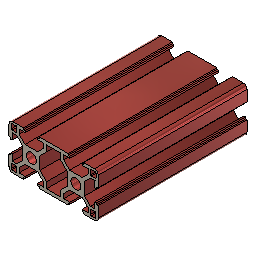
3060 Extrusion (Autodesk Fusion 360 design; units mm, degrees)
Autodesk Fusion 360 part; units mm, degrees
sketch "Sketch1" plane through (0, 0, 0) normal (0, 0, 1) x (1, 0, 0)
  circle A0 centre (10, 10) radius 2.5
  line L0 (13.9, 6.1) -> (6.1, 13.9) construction
  line L1 (0, 6.4) -> (0, 1.5)
  line L2 (4.5, 1.8) -> (6.9, 1.8)
  line L3 (3.5808, 4.5) -> (6.1, 7.0192)
  line L4 (4.5, 3.5808) -> (7.0192, 6.1)
  line L5 (0.5, 6.9) -> (0.5, 6.4)
  line L6 (0.5, 6.4) -> (0, 6.4)
  line L7 (6.9, 0) -> (6.4, 0) construction
  line L8 (6.4, 0) -> (6.4, 0.5)
  line L9 (6.4, 0.5) -> (6.9, 0.5)
  arc A1 (0, 1.5) -> (1.5, 0) centre (1.5, 1.5) ccw
  line L10 (1.8, 6.9) -> (0.5, 6.9)
  line L11 (1.8, 6.9) -> (1.8, 6.4)
  line L12 (1.8, 6.4) -> (1.8, 4.5)
  line L13 (3.5808, 4.5) -> (1.8, 4.5)
  line L14 (6.1, 10) -> (6.1, 7.0192)
  line L15 (7.0192, 6.1) -> (10, 6.1)
  line L16 (4.5, 1.8) -> (4.5, 3.5808)
  line L17 (6.9, 0.5) -> (6.9, 1.8)
  line L18 (1.5, 0) -> (6.4, 0)
  line L19 (6.4, 0) -> (6.9, 0)
  line L20 (0, 6.9) -> (0, 6.4)
  line L21 (10, 13.9) -> (10, 6.1) construction
  line L22 (13.9, 10) -> (6.1, 10) construction
  line L23 (20, 6.4) -> (19.5, 6.4)
  line L24 (19.5, 6.4) -> (19.5, 6.9)
  line L25 (19.5, 6.9) -> (18.2, 6.9)
  line L26 (18.2, 4.5) -> (18.2, 6.9)
  line L27 (18.2, 4.5) -> (16.4192, 4.5)
  line L28 (16.4192, 4.5) -> (13.9, 7.0192)
  line L29 (13.9, 7.0192) -> (13.9, 10)
  line L30 (15.5, 3.5808) -> (12.9808, 6.1)
  line L31 (15.5, 3.5808) -> (15.5, 1.8)
  line L32 (13.6, 1.8) -> (15.5, 1.8)
  line L33 (13.1, 1.8) -> (13.6, 1.8)
  line L34 (13.1, 1.8) -> (13.1, 0.5)
  line L35 (13.1, 0.5) -> (13.6, 0.5)
  line L36 (13.6, 0.5) -> (13.6, 0)
  line L37 (10, 6.1) -> (12.9808, 6.1)
  line L38 (13.6, 0) -> (18.5, 0)
  arc A2 (18.5, 0) -> (20, 1.5) centre (18.5, 1.5) ccw
  line L39 (20, 1.5) -> (20, 6.4)
  line L40 (13.6, 20) -> (13.6, 19.5)
  line L41 (13.6, 19.5) -> (13.1, 19.5)
  line L42 (13.1, 19.5) -> (13.1, 18.2)
  line L43 (15.5, 18.2) -> (13.1, 18.2)
  line L44 (15.5, 18.2) -> (15.5, 16.4192)
  line L45 (15.5, 16.4192) -> (12.9808, 13.9)
  line L46 (12.9808, 13.9) -> (10, 13.9)
  line L47 (16.4192, 15.5) -> (13.9, 12.9808)
  line L48 (16.4192, 15.5) -> (18.2, 15.5)
  line L49 (18.2, 13.6) -> (18.2, 15.5)
  line L50 (18.2, 13.1) -> (18.2, 13.6)
  line L51 (18.2, 13.1) -> (19.5, 13.1)
  line L52 (19.5, 13.1) -> (19.5, 13.6)
  line L53 (19.5, 13.6) -> (20, 13.6)
  line L54 (13.9, 10) -> (13.9, 12.9808)
  line L55 (20, 13.6) -> (20, 18.5)
  arc A3 (20, 18.5) -> (18.5, 20) centre (18.5, 18.5) ccw
  line L56 (18.5, 20) -> (13.6, 20)
  line L57 (0, 13.6) -> (0.5, 13.6)
  line L58 (0.5, 13.6) -> (0.5, 13.1)
  line L59 (0.5, 13.1) -> (1.8, 13.1)
  line L60 (1.8, 15.5) -> (1.8, 13.1)
  line L61 (1.8, 15.5) -> (3.5808, 15.5)
  line L62 (3.5808, 15.5) -> (6.1, 12.9808)
  line L63 (6.1, 12.9808) -> (6.1, 10)
  line L64 (4.5, 16.4192) -> (7.0192, 13.9)
  line L65 (4.5, 16.4192) -> (4.5, 18.2)
  line L66 (6.4, 18.2) -> (4.5, 18.2)
  line L67 (6.9, 18.2) -> (6.4, 18.2)
  line L68 (6.9, 18.2) -> (6.9, 19.5)
  line L69 (6.9, 19.5) -> (6.4, 19.5)
  line L70 (6.4, 19.5) -> (6.4, 20)
  line L71 (10, 13.9) -> (7.0192, 13.9)
  line L72 (6.4, 20) -> (1.5, 20)
  arc A4 (1.5, 20) -> (0, 18.5) centre (1.5, 18.5) ccw
  line L73 (0, 18.5) -> (0, 13.6)
  arc A5 (26, 1.5) -> (27.5, 0) centre (27.5, 1.5) ccw
  line L74 (41.5, 3.5808) -> (41.5, 1.8)
  line L75 (39.1, 19.5) -> (39.1, 18.2)
  line L76 (32.4, 20) -> (27.5, 20)
  line L77 (26, 6.9) -> (26, 6.4)
  line L78 (29.5808, 4.5) -> (32.1, 7.0192)
  line L79 (29.5808, 15.5) -> (32.1, 12.9808)
  line L80 (26, 13.6) -> (26.5, 13.6)
  line L81 (39.1, 0.5) -> (39.6, 0.5)
  line L82 (30.5, 16.4192) -> (30.5, 18.2)
  line L83 (27.8, 15.5) -> (27.8, 13.1)
  line L84 (36, 13.9) -> (36, 6.1) construction
  line L85 (32.4, 0) -> (32.4, 0.5)
  line L86 (39.6, 0.5) -> (39.6, 0)
  line L87 (32.1, 10) -> (32.1, 7.0192)
  line L88 (32.4, 19.5) -> (32.4, 20)
  line L89 (39.1, 1.8) -> (39.6, 1.8)
  line L90 (27.8, 6.9) -> (27.8, 6.4)
  line L91 (41.5, 16.4192) -> (38.9808, 13.9)
  line L92 (26.5, 13.1) -> (27.8, 13.1)
  line L93 (26.5, 6.4) -> (26, 6.4)
  line L94 (32.1, 12.9808) -> (32.1, 10)
  line L95 (27.5, 0) -> (32.4, 0)
  line L96 (32.9, 0.5) -> (32.9, 1.8)
  line L97 (32.9, 0) -> (32.4, 0) construction
  line L98 (30.5, 1.8) -> (30.5, 3.5808)
  line L99 (32.9, 19.5) -> (32.4, 19.5)
  line L100 (32.9, 18.2) -> (32.4, 18.2)
  line L101 (41.5, 18.2) -> (39.1, 18.2)
  line L102 (39.6, 19.5) -> (39.1, 19.5)
  line L103 (27.8, 6.9) -> (26.5, 6.9)
  line L104 (27.8, 15.5) -> (29.5808, 15.5)
  line L105 (36, 13.9) -> (33.0192, 13.9)
  line L106 (33.0192, 6.1) -> (36, 6.1)
  line L107 (41.5, 18.2) -> (41.5, 16.4192)
  line L108 (39.9, 10) -> (32.1, 10) construction
  line L109 (39.6, 1.8) -> (41.5, 1.8)
  line L110 (39.9, 6.1) -> (32.1, 13.9) construction
  line L111 (39.6, 0) -> (44.5, 0)
  line L112 (36, 6.1) -> (38.9808, 6.1)
  circle A6 centre (36, 10) radius 2.5
  line L113 (42.4192, 4.5) -> (39.9, 7.0192)
  line L114 (38.9808, 13.9) -> (36, 13.9)
  line L115 (41.5, 3.5808) -> (38.9808, 6.1)
  line L116 (39.9, 7.0192) -> (39.9, 10)
  line L117 (39.9, 10) -> (39.9, 12.9808)
  line L118 (30.5, 16.4192) -> (33.0192, 13.9)
  line L119 (42.4192, 15.5) -> (39.9, 12.9808)
  line L120 (26, 18.5) -> (26, 13.6)
  line L121 (39.6, 20) -> (39.6, 19.5)
  line L122 (32.4, 18.2) -> (30.5, 18.2)
  line L123 (26.5, 6.9) -> (26.5, 6.4)
  line L124 (39.1, 1.8) -> (39.1, 0.5)
  arc A7 (27.5, 20) -> (26, 18.5) centre (27.5, 18.5) ccw
  line L125 (44.5, 20) -> (39.6, 20)
  line L126 (26, 6.4) -> (26, 1.5)
  line L127 (30.5, 3.5808) -> (33.0192, 6.1)
  line L128 (32.4, 0) -> (32.9, 0)
  line L129 (32.4, 0.5) -> (32.9, 0.5)
  line L130 (29.5808, 4.5) -> (27.8, 4.5)
  line L131 (27.8, 6.4) -> (27.8, 4.5)
  line L132 (30.5, 1.8) -> (32.9, 1.8)
  line L133 (26.5, 13.6) -> (26.5, 13.1)
  line L134 (32.9, 18.2) -> (32.9, 19.5)
  line L135 (59.9, 6.1) -> (52.1, 13.9) construction
  circle A8 centre (56, 10) radius 2.5
  line L136 (56, 13.9) -> (56, 6.1) construction
  line L137 (66, 13.6) -> (66, 18.5)
  line L138 (61.5, 16.4192) -> (58.9808, 13.9)
  line L139 (59.9, 10) -> (59.9, 12.9808)
  line L140 (64.2, 13.1) -> (65.5, 13.1)
  line L141 (59.6, 20) -> (59.6, 19.5)
  line L142 (52.1, 12.9808) -> (52.1, 10)
  line L143 (59.1, 19.5) -> (59.1, 18.2)
  line L144 (64.2, 13.1) -> (64.2, 13.6)
  line L145 (64.2, 13.6) -> (64.2, 15.5)
  line L146 (59.9, 10) -> (52.1, 10) construction
  line L147 (65.5, 13.1) -> (65.5, 13.6)
  line L148 (64.5, 20) -> (59.6, 20)
  line L149 (49.5808, 15.5) -> (52.1, 12.9808)
  line L150 (52.4, 19.5) -> (52.4, 20)
  line L151 (62.4192, 15.5) -> (64.2, 15.5)
  line L152 (59.1, 0.5) -> (59.6, 0.5)
  line L153 (65.5, 13.6) -> (66, 13.6)
  line L154 (50.5, 16.4192) -> (53.0192, 13.9)
  line L155 (61.5, 18.2) -> (61.5, 16.4192)
  line L156 (53.0192, 6.1) -> (56, 6.1)
  line L157 (50.5, 16.4192) -> (50.5, 18.2)
  line L158 (52.4, 0.5) -> (52.9, 0.5)
  line L159 (59.1, 1.8) -> (59.6, 1.8)
  line L160 (49.5808, 4.5) -> (52.1, 7.0192)
  line L161 (50.5, 1.8) -> (50.5, 3.5808)
  line L162 (61.5, 3.5808) -> (61.5, 1.8)
  line L163 (56, 13.9) -> (53.0192, 13.9)
  line L164 (52.4, 0) -> (52.4, 0.5)
  line L165 (50.5, 3.5808) -> (53.0192, 6.1)
  line L166 (66, 1.5) -> (66, 6.4)
  line L167 (59.6, 1.8) -> (61.5, 1.8)
  arc A9 (66, 18.5) -> (64.5, 20) centre (64.5, 18.5) ccw
  line L168 (52.1, 10) -> (52.1, 7.0192)
  line L169 (64.2, 4.5) -> (62.4192, 4.5)
  line L170 (59.6, 19.5) -> (59.1, 19.5)
  line L171 (61.5, 18.2) -> (59.1, 18.2)
  line L172 (61.5, 3.5808) -> (58.9808, 6.1)
  line L173 (52.9, 0) -> (52.4, 0) construction
  line L174 (59.9, 7.0192) -> (59.9, 10)
  line L175 (52.4, 18.2) -> (50.5, 18.2)
  line L176 (59.6, 0.5) -> (59.6, 0)
  line L177 (52.9, 18.2) -> (52.4, 18.2)
  line L178 (66, 6.4) -> (65.5, 6.4)
  line L179 (56, 6.1) -> (58.9808, 6.1)
  line L180 (52.9, 18.2) -> (52.9, 19.5)
  line L181 (59.6, 0) -> (64.5, 0)
  line L182 (62.4192, 4.5) -> (59.9, 7.0192)
  arc A10 (64.5, 0) -> (66, 1.5) centre (64.5, 1.5) ccw
  line L183 (50.5, 1.8) -> (52.9, 1.8)
  line L184 (52.4, 20) -> (47.5, 20)
  line L185 (64.2, 4.5) -> (64.2, 6.9)
  line L186 (65.5, 6.4) -> (65.5, 6.9)
  line L187 (52.4, 0) -> (52.9, 0)
  line L188 (52.9, 19.5) -> (52.4, 19.5)
  line L189 (65.5, 6.9) -> (64.2, 6.9)
  line L190 (59.1, 1.8) -> (59.1, 0.5)
  line L191 (47.5, 0) -> (52.4, 0)
  line L192 (58.9808, 13.9) -> (56, 13.9)
  line L193 (62.4192, 15.5) -> (59.9, 12.9808)
  line L194 (52.9, 0.5) -> (52.9, 1.8)
  line L195 (44.5, 20) -> (47.5, 20)
  line L196 (44.5, 0) -> (47.5, 0)
  line L197 (41.5, 18.2) -> (42.8, 18.2) construction
  line L198 (42.8, 18.2) -> (49.2, 18.2)
  line L199 (49.2, 1.8) -> (42.8, 1.8)
  line L200 (42.4192, 15.5) -> (42.8, 15.8808)
  line L201 (49.5808, 15.5) -> (49.2, 15.8808)
  line L202 (49.5808, 4.5) -> (49.2, 4.1192)
  line L203 (42.4192, 4.5) -> (42.8, 4.1192)
  line L204 (42.8, 15.8808) -> (42.8, 18.2)
  line L205 (49.2, 18.2) -> (49.2, 15.8808)
  line L206 (49.2, 4.1192) -> (49.2, 1.8)
  line L207 (42.8, 1.8) -> (42.8, 4.1192)
  arc A11 (2.5, -14.9884) -> (0, -17.4884) centre (2.5, -17.4884) ccw
  circle A12 centre (15, -29.9884) radius 3.4
  line L208 (10.9, -15.9884) -> (10.9, -17.1884)
  line L209 (19.2444, -24.1884) -> (10.7556, -24.1884)
  line L210 (9.2, -25.744) -> (9.2, -34.2327)
  line L211 (10.7556, -35.7884) -> (19.2444, -35.7884)
  line L212 (20.8, -34.2327) -> (20.8, -25.744)
  line L213 (1, -25.8884) -> (2.2, -25.8884)
  line L214 (0, -24.7884) -> (0, -21.7384)
  line L215 (0, -24.7884) -> (1, -24.7884)
  line L216 (1, -25.8884) -> (1, -24.7884)
  line L217 (2.2, -25.8884) -> (2.2, -24.7884)
  line L218 (2.2, -24.7884) -> (2.2, -21.7384)
  line L219 (2.5, -14.9884) -> (9.8, -14.9884)
  line L220 (6.75, -17.1884) -> (10.9, -17.1884)
  line L221 (9.8, -15.9884) -> (10.9, -15.9884)
  line L222 (9.8, -15.9884) -> (9.8, -14.9884)
  line L223 (2.2, -21.7384) -> (5.1944, -21.7384)
  line L224 (6.75, -20.1827) -> (6.75, -17.1884)
  line L225 (0, -17.4884) -> (0, -21.7384)
  line L226 (10.7556, -24.1884) -> (6.75, -20.1827)
  line L227 (9.2, -25.744) -> (5.1944, -21.7384)
  line L228 (4.825, -20.1634) -> (2.075, -20.1634)
  line L229 (1.575, -19.6634) -> (1.575, -16.9134)
  line L230 (2.075, -16.4134) -> (4.825, -16.4134)
  line L231 (5.325, -16.9134) -> (5.325, -19.6634)
  arc A13 (2.075, -16.4134) -> (1.575, -16.9134) centre (2.075, -16.9134) ccw
  arc A14 (5.325, -16.9134) -> (4.825, -16.4134) centre (4.825, -16.9134) ccw
  arc A15 (4.825, -20.1634) -> (5.325, -19.6634) centre (4.825, -19.6634) ccw
  arc A16 (1.575, -19.6634) -> (2.075, -20.1634) centre (2.075, -19.6634) ccw
  line L232 (2.2, -38.2384) -> (2.2, -34.0884)
  line L233 (1, -34.0884) -> (2.2, -34.0884)
  line L234 (1, -35.1884) -> (1, -34.0884)
  line L235 (1, -35.1884) -> (0, -35.1884)
  line L236 (0, -42.4884) -> (0, -35.1884)
  arc A17 (0, -42.4884) -> (2.5, -44.9884) centre (2.5, -42.4884) ccw
  line L237 (2.5, -44.9884) -> (6.75, -44.9884)
  line L238 (9.8, -44.9884) -> (6.75, -44.9884)
  line L239 (9.8, -44.9884) -> (9.8, -43.9884)
  line L240 (10.9, -43.9884) -> (9.8, -43.9884)
  line L241 (10.9, -43.9884) -> (10.9, -42.7884)
  line L242 (10.9, -42.7884) -> (9.8, -42.7884)
  line L243 (9.8, -42.7884) -> (6.75, -42.7884)
  line L244 (6.75, -42.7884) -> (6.75, -39.794)
  line L245 (10.7556, -35.7884) -> (6.75, -39.794)
  line L246 (9.2, -34.2327) -> (5.1944, -38.2384)
  line L247 (5.1944, -38.2384) -> (2.2, -38.2384)
  arc A18 (1.425, -42.9134) -> (1.925, -43.4134) centre (1.925, -42.9134) ccw
  line L248 (1.425, -42.9134) -> (1.425, -40.1634)
  arc A19 (1.925, -39.6634) -> (1.425, -40.1634) centre (1.925, -40.1634) ccw
  line L249 (1.925, -39.6634) -> (4.675, -39.6634)
  arc A20 (5.175, -40.1634) -> (4.675, -39.6634) centre (4.675, -40.1634) ccw
  line L250 (5.175, -40.1634) -> (5.175, -42.9134)
  arc A21 (4.675, -43.4134) -> (5.175, -42.9134) centre (4.675, -42.9134) ccw
  line L251 (4.675, -43.4134) -> (1.925, -43.4134)
  line L252 (23.25, -42.7884) -> (19.1, -42.7884)
  line L253 (19.1, -43.9884) -> (19.1, -42.7884)
  line L254 (20.2, -43.9884) -> (19.1, -43.9884)
  line L255 (20.2, -43.9884) -> (20.2, -44.9884)
  line L256 (27.5, -44.9884) -> (20.2, -44.9884)
  arc A22 (27.5, -44.9884) -> (30, -42.4884) centre (27.5, -42.4884) ccw
  line L257 (30, -42.4884) -> (30, -38.2384)
  line L258 (30, -35.1884) -> (30, -38.2384)
  line L259 (30, -35.1884) -> (29, -35.1884)
  line L260 (29, -34.0884) -> (29, -35.1884)
  line L261 (29, -34.0884) -> (27.8, -34.0884)
  line L262 (27.8, -34.0884) -> (27.8, -35.1884)
  line L263 (27.8, -35.1884) -> (27.8, -38.2384)
  line L264 (27.8, -38.2384) -> (24.8056, -38.2384)
  line L265 (20.8, -34.2327) -> (24.8056, -38.2384)
  line L266 (19.2444, -35.7884) -> (23.25, -39.794)
  line L267 (23.25, -39.794) -> (23.25, -42.7884)
  arc A23 (27.925, -43.5634) -> (28.425, -43.0634) centre (27.925, -43.0634) ccw
  line L268 (27.925, -43.5634) -> (25.175, -43.5634)
  arc A24 (24.675, -43.0634) -> (25.175, -43.5634) centre (25.175, -43.0634) ccw
  line L269 (24.675, -43.0634) -> (24.675, -40.3134)
  arc A25 (25.175, -39.8134) -> (24.675, -40.3134) centre (25.175, -40.3134) ccw
  line L270 (25.175, -39.8134) -> (27.925, -39.8134)
  arc A26 (28.425, -40.3134) -> (27.925, -39.8134) centre (27.925, -40.3134) ccw
  line L271 (28.425, -40.3134) -> (28.425, -43.0634)
  line L272 (27.8, -21.7384) -> (27.8, -25.8884)
  line L273 (29, -25.8884) -> (27.8, -25.8884)
  line L274 (29, -24.7884) -> (29, -25.8884)
  line L275 (29, -24.7884) -> (30, -24.7884)
  line L276 (30, -17.4884) -> (30, -24.7884)
  arc A27 (30, -17.4884) -> (27.5, -14.9884) centre (27.5, -17.4884) ccw
  line L277 (27.5, -14.9884) -> (23.25, -14.9884)
  line L278 (20.2, -14.9884) -> (23.25, -14.9884)
  line L279 (20.2, -14.9884) -> (20.2, -15.9884)
  line L280 (19.1, -15.9884) -> (20.2, -15.9884)
  line L281 (19.1, -15.9884) -> (19.1, -17.1884)
  line L282 (19.1, -17.1884) -> (20.2, -17.1884)
  line L283 (20.2, -17.1884) -> (23.25, -17.1884)
  line L284 (23.25, -17.1884) -> (23.25, -20.1827)
  line L285 (19.2444, -24.1884) -> (23.25, -20.1827)
  line L286 (20.8, -25.744) -> (24.8056, -21.7384)
  line L287 (24.8056, -21.7384) -> (27.8, -21.7384)
  arc A28 (28.575, -17.0634) -> (28.075, -16.5634) centre (28.075, -17.0634) ccw
  line L288 (28.575, -17.0634) -> (28.575, -19.8134)
  arc A29 (28.075, -20.3134) -> (28.575, -19.8134) centre (28.075, -19.8134) ccw
  line L289 (28.075, -20.3134) -> (25.325, -20.3134)
  arc A30 (24.825, -19.8134) -> (25.325, -20.3134) centre (25.325, -19.8134) ccw
  line L290 (24.825, -19.8134) -> (24.825, -17.0634)
  arc A31 (25.325, -16.5634) -> (24.825, -17.0634) centre (25.325, -17.0634) ccw
  line L291 (25.325, -16.5634) -> (28.075, -16.5634)
  circle A32 centre (55, -29.9884) radius 3.4
  line L292 (59.1, -15.9884) -> (60.2, -15.9884)
  line L293 (59.1, -43.9884) -> (59.1, -42.7884)
  line L294 (50.9, -43.9884) -> (50.9, -42.7884)
  line L295 (50.9, -42.7884) -> (49.8, -42.7884)
  line L296 (49.8, -44.9884) -> (49.8, -43.9884)
  line L297 (60.8, -34.2327) -> (60.8, -25.744)
  line L298 (49.8, -15.9884) -> (49.8, -14.9884)
  line L299 (50.9, -15.9884) -> (50.9, -17.1884)
  line L300 (60.2, -17.1884) -> (63.25, -17.1884)
  line L301 (50.9, -43.9884) -> (49.8, -43.9884)
  line L302 (50.7556, -35.7884) -> (59.2444, -35.7884)
  line L303 (59.2444, -24.1884) -> (63.25, -20.1827)
  line L304 (59.1, -15.9884) -> (59.1, -17.1884)
  line L305 (59.2444, -35.7884) -> (63.25, -39.794)
  line L306 (60.2, -43.9884) -> (59.1, -43.9884)
  line L307 (49.8, -15.9884) -> (50.9, -15.9884)
  line L308 (59.1, -17.1884) -> (60.2, -17.1884)
  line L309 (60.2, -14.9884) -> (60.2, -15.9884)
  line L310 (60.2, -43.9884) -> (60.2, -44.9884)
  line L311 (59.2444, -24.1884) -> (50.7556, -24.1884)
  line L312 (63.25, -42.7884) -> (59.1, -42.7884)
  arc A33 (41.575, -19.6634) -> (42.075, -20.1634) centre (42.075, -19.6634) ccw
  line L313 (40, -17.4884) -> (40, -21.7384)
  line L314 (42.2, -24.7884) -> (42.2, -21.7384)
  line L315 (40, -24.7884) -> (41, -24.7884)
  line L316 (67.5, -44.9884) -> (60.2, -44.9884)
  line L317 (41, -25.8884) -> (42.2, -25.8884)
  arc A34 (42.075, -16.4134) -> (41.575, -16.9134) centre (42.075, -16.9134) ccw
  line L318 (44.825, -20.1634) -> (42.075, -20.1634)
  line L319 (42.2, -25.8884) -> (42.2, -24.7884)
  arc A35 (45.325, -16.9134) -> (44.825, -16.4134) centre (44.825, -16.9134) ccw
  line L320 (60.8, -34.2327) -> (64.8056, -38.2384)
  arc A36 (42.5, -14.9884) -> (40, -17.4884) centre (42.5, -17.4884) ccw
  line L321 (40, -24.7884) -> (40, -21.7384)
  line L322 (60.8, -25.744) -> (64.8056, -21.7384)
  line L323 (45.325, -16.9134) -> (45.325, -19.6634)
  line L324 (60.2, -14.9884) -> (63.25, -14.9884)
  line L325 (42.5, -14.9884) -> (49.8, -14.9884)
  line L326 (50.7556, -24.1884) -> (46.75, -20.1827)
  line L327 (41.575, -19.6634) -> (41.575, -16.9134)
  line L328 (49.8, -42.7884) -> (46.75, -42.7884)
  line L329 (46.75, -17.1884) -> (50.9, -17.1884)
  line L330 (49.2, -25.744) -> (45.1944, -21.7384)
  line L331 (46.75, -20.1827) -> (46.75, -17.1884)
  line L332 (49.8, -44.9884) -> (46.75, -44.9884)
  line L333 (50.7556, -35.7884) -> (46.75, -39.794)
  arc A37 (44.825, -20.1634) -> (45.325, -19.6634) centre (44.825, -19.6634) ccw
  line L334 (42.075, -16.4134) -> (44.825, -16.4134)
  line L335 (63.25, -39.794) -> (63.25, -42.7884)
  line L336 (41, -25.8884) -> (41, -24.7884)
  line L337 (49.2, -25.744) -> (49.2, -34.2327)
  line L338 (42.2, -21.7384) -> (45.1944, -21.7384)
  line L339 (42.2, -38.2384) -> (42.2, -34.0884)
  line L340 (41.425, -42.9134) -> (41.425, -40.1634)
  arc A38 (45.175, -40.1634) -> (44.675, -39.6634) centre (44.675, -40.1634) ccw
  arc A39 (41.425, -42.9134) -> (41.925, -43.4134) centre (41.925, -42.9134) ccw
  line L341 (41, -35.1884) -> (40, -35.1884)
  arc A40 (41.925, -39.6634) -> (41.425, -40.1634) centre (41.925, -40.1634) ccw
  line L342 (41.925, -39.6634) -> (44.675, -39.6634)
  line L343 (45.175, -40.1634) -> (45.175, -42.9134)
  line L344 (49.2, -34.2327) -> (45.1944, -38.2384)
  line L345 (67.5, -14.9884) -> (63.25, -14.9884)
  arc A41 (44.675, -43.4134) -> (45.175, -42.9134) centre (44.675, -42.9134) ccw
  arc A42 (40, -42.4884) -> (42.5, -44.9884) centre (42.5, -42.4884) ccw
  line L346 (41, -35.1884) -> (41, -34.0884)
  line L347 (41, -34.0884) -> (42.2, -34.0884)
  line L348 (42.5, -44.9884) -> (46.75, -44.9884)
  line L349 (63.25, -17.1884) -> (63.25, -20.1827)
  line L350 (40, -42.4884) -> (40, -35.1884)
  line L351 (46.75, -42.7884) -> (46.75, -39.794)
  line L352 (45.1944, -38.2384) -> (42.2, -38.2384)
  line L353 (44.675, -43.4134) -> (41.925, -43.4134)
  line L354 (90.2, -43.9884) -> (89.1, -43.9884)
  arc A43 (95.175, -39.8134) -> (94.675, -40.3134) centre (95.175, -40.3134) ccw
  circle A44 centre (85, -29.9884) radius 3.4
  arc A45 (98.425, -40.3134) -> (97.925, -39.8134) centre (97.925, -40.3134) ccw
  line L355 (97.925, -43.5634) -> (95.175, -43.5634)
  line L356 (79.8, -44.9884) -> (79.8, -43.9884)
  line L357 (97.8, -38.2384) -> (94.8056, -38.2384)
  line L358 (100, -17.4884) -> (100, -24.7884)
  line L359 (90.2, -14.9884) -> (93.25, -14.9884)
  line L360 (89.1, -15.9884) -> (89.1, -17.1884)
  line L361 (76.75, -42.7884) -> (76.75, -39.794)
  line L362 (97.8, -34.0884) -> (97.8, -35.1884)
  arc A46 (97.5, -44.9884) -> (100, -42.4884) centre (97.5, -42.4884) ccw
  line L363 (80.9, -43.9884) -> (80.9, -42.7884)
  line L364 (89.1, -43.9884) -> (89.1, -42.7884)
  line L365 (94.675, -43.0634) -> (94.675, -40.3134)
  line L366 (95.175, -39.8134) -> (97.925, -39.8134)
  line L367 (80.9, -42.7884) -> (79.8, -42.7884)
  line L368 (93.25, -39.794) -> (93.25, -42.7884)
  line L369 (98.425, -40.3134) -> (98.425, -43.0634)
  line L370 (90.2, -43.9884) -> (90.2, -44.9884)
  line L371 (100, -42.4884) -> (100, -38.2384)
  line L372 (100, -35.1884) -> (100, -38.2384)
  line L373 (100, -35.1884) -> (99, -35.1884)
  line L374 (90.8, -34.2327) -> (94.8056, -38.2384)
  line L375 (97.5, -44.9884) -> (90.2, -44.9884)
  line L376 (99, -34.0884) -> (99, -35.1884)
  arc A47 (95.325, -16.5634) -> (94.825, -17.0634) centre (95.325, -17.0634) ccw
  line L377 (90.8, -34.2327) -> (90.8, -25.744)
  line L378 (80.7556, -35.7884) -> (76.75, -39.794)
  line L379 (80.7556, -24.1884) -> (76.75, -20.1827)
  arc A48 (98.075, -20.3134) -> (98.575, -19.8134) centre (98.075, -19.8134) ccw
  line L380 (98.075, -20.3134) -> (95.325, -20.3134)
  line L381 (79.2, -25.744) -> (75.1944, -21.7384)
  line L382 (89.2444, -24.1884) -> (80.7556, -24.1884)
  line L383 (79.8, -42.7884) -> (76.75, -42.7884)
  line L384 (89.1, -17.1884) -> (90.2, -17.1884)
  line L385 (90.2, -17.1884) -> (93.25, -17.1884)
  line L386 (72.5, -14.9884) -> (79.8, -14.9884)
  line L387 (79.2, -34.2327) -> (75.1944, -38.2384)
  line L388 (97.8, -21.7384) -> (97.8, -25.8884)
  line L389 (99, -25.8884) -> (97.8, -25.8884)
  line L390 (94.825, -19.8134) -> (94.825, -17.0634)
  line L391 (79.8, -44.9884) -> (76.75, -44.9884)
  line L392 (90.8, -25.744) -> (94.8056, -21.7384)
  line L393 (79.8, -15.9884) -> (80.9, -15.9884)
  arc A49 (100, -17.4884) -> (97.5, -14.9884) centre (97.5, -17.4884) ccw
  line L394 (89.1, -15.9884) -> (90.2, -15.9884)
  line L395 (79.2, -25.744) -> (79.2, -34.2327)
  line L396 (72.5, -44.9884) -> (76.75, -44.9884)
  line L397 (93.25, -17.1884) -> (93.25, -20.1827)
  line L398 (80.9, -15.9884) -> (80.9, -17.1884)
  line L399 (79.8, -15.9884) -> (79.8, -14.9884)
  line L400 (99, -24.7884) -> (100, -24.7884)
  line L401 (94.8056, -21.7384) -> (97.8, -21.7384)
  line L402 (95.325, -16.5634) -> (98.075, -16.5634)
  line L403 (90.2, -14.9884) -> (90.2, -15.9884)
  arc A50 (94.825, -19.8134) -> (95.325, -20.3134) centre (95.325, -19.8134) ccw
  line L404 (98.575, -17.0634) -> (98.575, -19.8134)
  line L405 (89.2444, -24.1884) -> (93.25, -20.1827)
  line L406 (76.75, -17.1884) -> (80.9, -17.1884)
  arc A51 (98.575, -17.0634) -> (98.075, -16.5634) centre (98.075, -17.0634) ccw
  line L407 (97.5, -14.9884) -> (93.25, -14.9884)
  line L408 (99, -24.7884) -> (99, -25.8884)
  line L409 (80.7556, -35.7884) -> (89.2444, -35.7884)
  line L410 (97.8, -35.1884) -> (97.8, -38.2384)
  arc A52 (94.675, -43.0634) -> (95.175, -43.5634) centre (95.175, -43.0634) ccw
  line L411 (89.2444, -35.7884) -> (93.25, -39.794)
  arc A53 (97.925, -43.5634) -> (98.425, -43.0634) centre (97.925, -43.0634) ccw
  line L412 (93.25, -42.7884) -> (89.1, -42.7884)
  line L413 (80.9, -43.9884) -> (79.8, -43.9884)
  line L414 (99, -34.0884) -> (97.8, -34.0884)
  line L415 (76.75, -20.1827) -> (76.75, -17.1884)
  line L416 (67.5, -14.9884) -> (72.5, -14.9884)
  line L417 (75.1944, -21.7384) -> (74.75, -21.294)
  line L418 (64.8056, -21.7384) -> (65.25, -21.294)
  line L419 (65.25, -17.1884) -> (74.75, -17.1884)
  line L420 (65.25, -17.1884) -> (65.25, -21.294)
  line L421 (74.75, -17.1884) -> (74.75, -21.294)
  line L422 (65.25, -42.7884) -> (65.25, -38.6827)
  line L423 (67.5, -44.9884) -> (72.5, -44.9884)
  line L424 (74.75, -42.7884) -> (74.75, -38.6827)
  line L425 (74.75, -42.7884) -> (65.25, -42.7884)
  line L426 (64.8056, -38.2384) -> (65.25, -38.6827)
  line L427 (75.1944, -38.2384) -> (74.75, -38.6827)
  point P0 (10, 10)
  point P1 (36, 10)
  point P2 (56, 10)
  point P3 (0, -14.9884)
  point P4 (30, -14.9884)
  point P5 (0, -44.9884)
  point P6 (15, -29.9884)
  point P7 (15, -29.9884)
  point P8 (15, -29.9884)
  point P9 (15, -29.9884)
  point P10 (15, -29.9884)
  point P11 (15, -29.9884)
  point P12 (15, -29.9884)
  point P13 (1.575, -20.1634)
  point P14 (1.575, -16.4134)
  point P15 (5.325, -16.4134)
  point P16 (3.45, -18.2884)
  point P17 (45.325, -16.4134)
  point P18 (43.45, -18.2884)
  point P19 (55, -29.9884)
  point P20 (41.575, -20.1634)
  point P21 (41.575, -16.4134)
  point P22 (55, -29.9884)
  point P23 (55, -29.9884)
  point P24 (55, -29.9884)
  point P25 (40, -44.9884)
  point P26 (40, -14.9884)
  point P27 (70, -14.9884)
  point P28 (55, -29.9884)
  point P29 (55, -29.9884)
  point P30 (55, -29.9884)
  point P31 (85, -29.9884)
  point P32 (73.45, -18.2884)
  point P33 (85, -29.9884)
  point P34 (71.575, -20.1634)
  point P35 (75.325, -16.4134)
  point P36 (70, -44.9884)
  point P37 (70, -14.9884)
  point P38 (100, -14.9884)
  point P39 (85, -29.9884)
  point P40 (85, -29.9884)
  point P41 (71.575, -16.4134)
  point P42 (85, -29.9884)
  point P43 (85, -29.9884)
  point P44 (85, -29.9884)
  dimension "d3" = 5
  dimension "d6" = 6.9
  dimension "d7" = 6.9
  dimension "d14" = 6.4
  dimension "d22" = 0.5
  dimension "d23" = 0.5
  dimension "d24" = 0.5
  dimension "d25" = 0.5
  dimension "d26" = 1.5
  dimension "d28" = 360
  dimension "d30" = 360
  dimension "d31" = 5
  dimension "d32" = 0.5
  dimension "d33" = 0.5
  dimension "d34" = 0.5
  dimension "d35" = 0.5
  dimension "d36" = 1.5
  dimension "d39" = 5
  dimension "d42" = 0.5
  dimension "d43" = 0.5
  dimension "d45" = 1.3
  dimension "d47" = 6.4
  dimension "d73" = 30
  dimension "d74" = 30
  dimension "d75" = 2.5
  dimension "d76" = 6.8
  dimension "d90" = 3.75
  dimension "d91" = 3.75
  dimension "d92" = 0.5
  dimension "d94" = 360
  dimension "d96" = 360
  dimension "d97" = 30
  dimension "d98" = 30
  dimension "d99" = 2.5
  dimension "d100" = 6.8
  dimension "d101" = 2.2
  dimension "d102" = 3.75
  dimension "d103" = 3.75
  dimension "d104" = 0.5
  dimension "d107" = 30
  dimension "d108" = 30
  dimension "d110" = 6.8
  dimension "d111" = 2.2
  dimension "d112" = 3.75
  dimension "d113" = 3.75
  dimension "d115" = 2
  dimension "d116" = 2
  dimension "d117" = 2
  dimension "d118" = 2
  constraint horizontal L18
  constraint coincident L0 P0
  constraint coincident P0 A0.centre
  constraint vertical L1
  constraint vertical L11
  constraint horizontal L2
  constraint vertical L5
  constraint horizontal L6
  constraint horizontal L7
  constraint vertical L8
  constraint horizontal L9
  constraint tangent L1 A1
  constraint tangent A1 L18
  constraint perpendicular L15 L21
  constraint perpendicular L14 L22
  constraint horizontal L95
  constraint coincident P1 L110
  constraint coincident P1 A6.centre
  constraint vertical L126
  constraint vertical L90
  constraint horizontal L132
  constraint vertical L123
  constraint horizontal L93
  constraint horizontal L97
  constraint vertical L85
  constraint horizontal L129
  constraint tangent A5 L126
  constraint tangent A5 L95
  constraint perpendicular L84 L106
  constraint perpendicular L87 L108
  constraint horizontal L191
  constraint coincident P2 L135
  constraint coincident P2 A8.centre
  constraint horizontal L183
  constraint horizontal L173
  constraint vertical L164
  constraint horizontal L158
  constraint perpendicular L136 L156
  constraint perpendicular L146 L168
  constraint perpendicular L107 L195
  constraint parallel L191 L196
  constraint perpendicular L107 L197
  constraint horizontal L198
  constraint horizontal L199
  constraint parallel L119 L200
  constraint perpendicular L200 L201
  constraint perpendicular L201 L202
  constraint perpendicular L202 L203
  constraint vertical L204
  constraint vertical L205
  constraint vertical L206
  constraint vertical L207
  constraint horizontal L219
  constraint coincident P3 L219
  constraint tangent A11 L219
  constraint coincident P4 L219
  constraint coincident P12 P11
  constraint horizontal L209
  constraint perpendicular L209 L210
  constraint parallel L209 L211
  constraint parallel L210 L212
  constraint horizontal L213
  constraint horizontal L215
  constraint tangent A11 L225
  constraint horizontal L228
  constraint perpendicular L228 L229
  constraint parallel L228 L230
  constraint parallel L229 L231
  constraint coincident P14 L229
  constraint coincident P14 L230
  constraint tangent L229 A13
  constraint tangent L230 A13
  constraint coincident P15 L230
  constraint coincident P15 L231
  constraint tangent L230 A14
  constraint tangent L231 A14
  constraint equal A13 A14
  constraint tangent L228 A15
  constraint tangent L231 A15
  constraint equal A13 A15
  constraint coincident P13 L228
  constraint coincident P13 L229
  constraint tangent L228 A16
  constraint tangent L229 A16
  constraint equal A13 A16
  constraint horizontal L325
  constraint coincident P26 L325
  constraint tangent A36 L325
  constraint coincident P37 L325
  constraint coincident P30 P29
  constraint horizontal L311
  constraint perpendicular L311 L337
  constraint parallel L302 L311
  constraint parallel L297 L337
  constraint horizontal L317
  constraint horizontal L315
  constraint tangent L313 A36
  constraint horizontal L318
  constraint perpendicular L318 L327
  constraint parallel L318 L334
  constraint parallel L323 L327
  constraint coincident P21 L327
  constraint coincident P21 L334
  constraint tangent A34 L327
  constraint tangent A34 L334
  constraint coincident P17 L334
  constraint coincident P17 L323
  constraint tangent A35 L334
  constraint tangent A35 L323
  constraint equal A34 A35
  constraint tangent L318 A37
  constraint tangent L323 A37
  constraint equal A34 A37
  constraint coincident P20 L318
  constraint coincident P20 L327
  constraint tangent A33 L318
  constraint tangent A33 L327
  constraint equal A33 A34
  constraint horizontal L386
  constraint coincident P37 L386
  constraint coincident P38 L386
  constraint coincident P44 P43
  constraint horizontal L382
  constraint perpendicular L382 L395
  constraint parallel L382 L409
  constraint parallel L377 L395
  constraint parallel L386 L416
  constraint parallel L381 L417
  constraint perpendicular L417 L418
  constraint vertical L420
  constraint vertical L421
  constraint vertical L422
  constraint parallel L396 L423
  constraint vertical L424
  constraint perpendicular L422 L425
  constraint parallel L320 L426
  constraint perpendicular L426 L427
  measures "d3" diameter of A0
  measures "d6" distance of origin L7.start
  measures "d7" distance of origin L20.start
  measures "d14" distance of origin L1.start
  measures "d22" distance of L20.start L5.start
  measures "d23" distance of L20.start L1.start
  measures "d24" distance of L7.start L7.end
  measures "d25" distance of L7.start L9.end
  measures "d26" radius of A1
  measures "d31" diameter of A6
  measures "d32" distance of L77.start L103.end
  measures "d33" distance of L77.start L77.end
  measures "d34" distance of L97.start L85.start
  measures "d35" distance of L97.start L96.start
  measures "d36" radius of A5
  measures "d39" diameter of A8
  measures "d42" distance of L173.start L164.start
  measures "d43" distance of L173.start L158.end
  measures "d45" distance of L101.start L197.end
  measures "d47" distance of L197.end L198.end
  measures "d73" distance of P3 P4
  measures "d74" distance of P3 P5
  measures "d75" radius of A11
  measures "d76" diameter of A12
  measures "d90" distance of P14 P15
  measures "d91" distance of P13 P14
  measures "d92" radius of A13
  measures "d97" distance of P26 P37
  measures "d98" distance of P25 P26
  measures "d99" radius of A36
  measures "d100" diameter of A32
  measures "d101" distance of L325 L329
  measures "d102" distance of P17 P21
  measures "d103" distance of P20 P21
  measures "d104" radius of A34
  measures "d107" distance of P37 P38
  measures "d108" distance of P36 P37
  measures "d110" diameter of A44
  measures "d111" distance of L386 L406
  measures "d112" distance of P35 P41
  measures "d113" distance of P34 P41
  measures "d115" distance of L300.end L419.start
  measures "d116" distance of L406.start L419.end
  measures "d117" distance of L312.start L422.start
  measures "d118" distance of L361.start L424.start
extrude "Extrude1" add sketch "Sketch1" along normal blind 100 makes body 1 at (12.4876, 9.7511, 33.3333) makes body 2 at (38.4876, 9.7511, 33.3333) makes body 3 at (18.3831, -30.3269, 33.3333) makes body 4 at (58.3831, -30.3269, 33.3333)
hidden bodies 1 2 3
equation "d7 = 10 mm - 3.1 mm"
equation "d14 = 10 mm - 3.6 mm"
named bodies: "2020 Extrusion", "2040 Extrusion", "3030 Extrusion", "3060 Extrusion"
